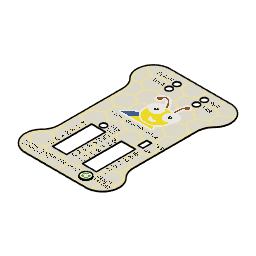
tiny-scarab-v0.2-membrane (Autodesk Fusion 360 design; units mm, degrees)
Autodesk Fusion 360 part; units mm, degrees
sketch "sketch 195" plane through (0, 0, 0) normal (0, 0, 1) x (1, 0, 0)
  arc A0 (79.75, -17.495) -> (71.5357, -37.0433) centre (79.75, -28.995) ccw construction
  line L0 (79.75, -17.495) -> (110.75, -17.495) construction
  arc A1 (118.9643, -37.0433) -> (110.75, -17.495) centre (110.75, -28.995) ccw construction
  arc A2 (118.9643, -37.0433) -> (117.25, -41.2424) centre (123.25, -41.2424) ccw construction
  line L1 (117.25, -41.2424) -> (117.25, -73.7476) construction
  arc A3 (117.25, -73.7476) -> (118.9643, -77.9467) centre (123.25, -73.7476) ccw construction
  arc A4 (110.75, -97.495) -> (118.9643, -77.9467) centre (110.75, -85.995) ccw construction
  line L2 (79.75, -97.495) -> (110.75, -97.495) construction
  arc A5 (71.5357, -77.9467) -> (79.75, -97.495) centre (79.75, -85.995) ccw construction
  arc A6 (71.5357, -77.9467) -> (73.25, -73.7476) centre (67.25, -73.7476) ccw construction
  line L3 (73.25, -41.2424) -> (73.25, -73.7476) construction
  arc A7 (73.25, -41.2424) -> (71.5357, -37.0433) centre (67.25, -41.2424) ccw construction
  arc A8 (114.25, -73.7476) -> (116.8214, -80.0462) centre (123.25, -73.7476) ccw
  arc A9 (110.75, -94.495) -> (116.8214, -80.0462) centre (110.75, -85.995) ccw
  line L4 (79.75, -94.495) -> (110.75, -94.495)
  arc A10 (73.6786, -80.0462) -> (79.75, -94.495) centre (79.75, -85.995) ccw
  arc A11 (73.6786, -80.0462) -> (76.25, -73.7476) centre (67.25, -73.7476) ccw
  line L5 (76.25, -41.2424) -> (76.25, -73.7476)
  arc A12 (76.25, -41.2424) -> (73.6786, -34.9438) centre (67.25, -41.2424) ccw
  arc A13 (79.75, -20.495) -> (73.6786, -34.9438) centre (79.75, -28.995) ccw
  line L6 (79.75, -20.495) -> (110.75, -20.495)
  arc A14 (116.8214, -34.9438) -> (110.75, -20.495) centre (110.75, -28.995) ccw
  arc A15 (116.8214, -34.9438) -> (114.25, -41.2424) centre (123.25, -41.2424) ccw
  line L7 (114.25, -41.2424) -> (114.25, -73.7476)
extrude "Extrude1" add sketch "sketch 195" along normal blind 0.2 makes body 1
sketch "sketch 402" plane through (0, 0, 0) normal (0, 0, 1) x (1, 0, 0)
  circle A0 centre (88.25, -25.495) radius 1.535
  circle A1 centre (88.25, -29.495) radius 1.535
  circle A2 centre (102.25, -25.495) radius 1.535
  circle A3 centre (102.25, -29.495) radius 1.535
  circle A4 centre (87.75, -62.495) radius 1.535
extrude "Extrude2" cut sketch "sketch 402" along normal through all bodies 1
sketch "sketch 509" plane through (0, 0, 0) normal (0, 0, 1) x (1, 0, 0)
  circle A0 centre (83.25, -26.495) radius 1.5 construction
  circle A1 centre (83.25, -34.995) radius 1.5 construction
  circle A2 centre (107.25, -26.495) radius 1.5 construction
  circle A3 centre (105.75, -89.495) radius 1.5 construction
  line L0 (105.43, -58.075) -> (107.93, -58.075)
  line L1 (105.43, -62.575) -> (105.43, -58.075)
  line L2 (107.93, -62.575) -> (105.43, -62.575)
  line L3 (107.93, -58.075) -> (107.93, -62.575)
  circle A4 centre (105.75, -89.495) radius 2.5
extrude "Extrude3" cut sketch "sketch 509" along normal through all contours L0 L1 L2 L3 bodies 1
sketch "sketch 540" plane through (0, 0, 0) normal (0, 0, 1) x (1, 0, 0)
  line L0 (91.23, -84.882) -> (84.03, -84.882)
  line L1 (84.03, -84.882) -> (84.03, -64.882)
  line L2 (84.03, -64.882) -> (91.23, -64.882)
  line L3 (91.23, -64.882) -> (91.23, -84.882)
  line L4 (99.27, -64.882) -> (106.47, -64.882)
  line L5 (99.27, -84.882) -> (99.27, -64.882)
  line L6 (106.47, -84.882) -> (99.27, -84.882)
  line L7 (106.47, -64.882) -> (106.47, -84.882)
extrude "Extrude4" cut sketch "sketch 540" along normal through all bodies 1
extrude "Extrude5" add sketch "sketch 509" along normal blind 0.5 separate body contours A4 makes body 2
